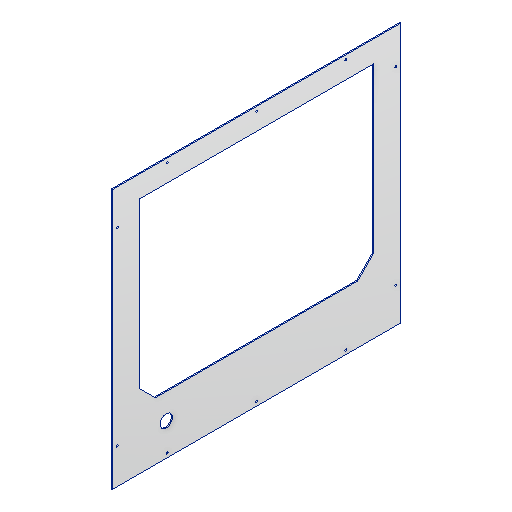
# Autodesk Inventor part: Front Panel
Saved by Autodesk Inventor 2023.2 (Build 272271000, 271)
## iProperties
Created: 2023-02-06
Part Number: Front Panel
Material: Aluminum 6061
Document SubType Name: Modeling
Designer: remop
Density: 2.7 g/cm^3
Appearance: Aluminum - Flat
Author: remop
Autodesk Inventor part; units mm, degrees
ref_plane "YZ Plane" through (0, 0, 0) normal (1, 0, 0) x (0, 1, 0)
ref_plane "XZ Plane" through (0, 0, 0) normal (0, 1, 0) x (-1, 0, 0)
ref_plane "XY Plane" through (0, 0, 0) normal (0, 0, 1) x (1, 0, 0)
sketch "Sketch1" plane through (0, 0, 0) normal (1, 0, 0) x (0, 1, 0)
  line L0 (465, 411) -> (465, -123) projected
  line L1 (465, -123) -> (-15, -123) projected
  line L2 (-15, -123) -> (-15, 411) projected
  line L3 (-15, 411) -> (465, 411) projected
  circle A0 centre (400, -113.5) radius 1.75 projected
  circle A1 centre (50, 401.5) radius 1.75 projected
  circle A2 centre (400, 401.5) radius 1.75 projected
  circle A3 centre (-7.5, -21) radius 1.75 projected
  circle A4 centre (-7.5, 144) radius 1.75 projected
  circle A5 centre (-7.5, 309) radius 1.75 projected
  circle A6 centre (457.5, 144) radius 1.75 projected
  circle A7 centre (457.5, -21) radius 1.75 projected
  circle A8 centre (457.5, 309) radius 1.75 projected
  circle A9 centre (50, -113.5) radius 1.75 projected
  circle A10 centre (408.5, -78.0001) radius 1.75 projected
  circle A11 centre (415.5, -88.0001) radius 1.75 projected
  circle A12 centre (408.5, -88.0001) radius 1.75 projected
  circle A13 centre (415.5, -78.0001) radius 1.75 projected
  line L4 (32, 375.1132) -> (32, 380.8868) projected
  line L5 (32, 380.8868) -> (27, 383.7735) projected
  line L6 (27, 383.7735) -> (22, 380.8868) projected
  line L7 (22, 380.8868) -> (22, 375.1132) projected
  line L8 (22, 375.1132) -> (27, 372.2265) projected
  line L9 (27, 372.2265) -> (32, 375.1132) projected
  line L10 (44.5, 367.8964) -> (44.5, 362.1229) projected
  line L11 (44.5, 362.1229) -> (49.5, 359.2361) projected
  line L12 (49.5, 359.2361) -> (54.5, 362.1229) projected
  line L13 (54.5, 362.1229) -> (54.5, 367.8964) projected
  line L14 (54.5, 367.8964) -> (49.5, 370.7831) projected
  line L15 (49.5, 370.7831) -> (44.5, 367.8964) projected
  line L16 (39.5, 336.1229) -> (39.5, 341.8964) projected
  line L17 (39.5, 341.8964) -> (34.5, 344.7831) projected
  line L18 (34.5, 344.7831) -> (29.5, 341.8964) projected
  line L19 (29.5, 341.8964) -> (29.5, 336.1229) projected
  line L20 (29.5, 336.1229) -> (34.5, 333.2361) projected
  line L21 (34.5, 333.2361) -> (39.5, 336.1229) projected
  line L22 (12, 331.7735) -> (7, 328.8868) projected
  line L23 (7, 328.8868) -> (7, 323.1132) projected
  line L24 (7, 323.1132) -> (12, 320.2265) projected
  line L25 (12, 320.2265) -> (17, 323.1132) projected
  line L26 (17, 323.1132) -> (17, 328.8868) projected
  line L27 (17, 328.8868) -> (12, 331.7735) projected
  line L28 (54.5, 315.8964) -> (49.5, 318.7831) projected
  line L29 (49.5, 318.7831) -> (44.5, 315.8964) projected
  line L30 (44.5, 315.8964) -> (44.5, 310.1229) projected
  line L31 (44.5, 310.1229) -> (49.5, 307.2361) projected
  line L32 (49.5, 307.2361) -> (54.5, 310.1229) projected
  line L33 (54.5, 310.1229) -> (54.5, 315.8964) projected
  line L34 (14.5, 310.1229) -> (19.5, 307.2361) projected
  line L35 (19.5, 307.2361) -> (24.5, 310.1229) projected
  line L36 (24.5, 310.1229) -> (24.5, 315.8964) projected
  line L37 (24.5, 315.8964) -> (19.5, 318.7831) projected
  line L38 (19.5, 318.7831) -> (14.5, 315.8964) projected
  line L39 (14.5, 315.8964) -> (14.5, 310.1229) projected
  line L40 (14.5, 284.1229) -> (19.5, 281.2361) projected
  line L41 (19.5, 281.2361) -> (24.5, 284.1229) projected
  line L42 (24.5, 284.1229) -> (24.5, 289.8964) projected
  line L43 (24.5, 289.8964) -> (19.5, 292.7831) projected
  line L44 (19.5, 292.7831) -> (14.5, 289.8964) projected
  line L45 (14.5, 289.8964) -> (14.5, 284.1229) projected
  line L46 (32, 276.8868) -> (27, 279.7735) projected
  line L47 (27, 279.7735) -> (22, 276.8868) projected
  line L48 (22, 276.8868) -> (22, 271.1132) projected
  line L49 (22, 271.1132) -> (27, 268.2265) projected
  line L50 (27, 268.2265) -> (32, 271.1132) projected
  line L51 (32, 271.1132) -> (32, 276.8868) projected
  line L52 (54.5, 263.8964) -> (49.5, 266.7831) projected
  line L53 (49.5, 266.7831) -> (44.5, 263.8964) projected
  line L54 (44.5, 263.8964) -> (44.5, 258.1229) projected
  line L55 (44.5, 258.1229) -> (49.5, 255.2361) projected
  line L56 (49.5, 255.2361) -> (54.5, 258.1229) projected
  line L57 (54.5, 258.1229) -> (54.5, 263.8964) projected
  line L58 (12, 253.7735) -> (7, 250.8868) projected
  line L59 (7, 250.8868) -> (7, 245.1132) projected
  line L60 (7, 245.1132) -> (12, 242.2265) projected
  line L61 (12, 242.2265) -> (17, 245.1132) projected
  line L62 (17, 245.1132) -> (17, 250.8868) projected
  line L63 (17, 250.8868) -> (12, 253.7735) projected
  line L64 (32, 224.8868) -> (27, 227.7735) projected
  line L65 (27, 227.7735) -> (22, 224.8868) projected
  line L66 (22, 224.8868) -> (22, 219.1132) projected
  line L67 (22, 219.1132) -> (27, 216.2265) projected
  line L68 (27, 216.2265) -> (32, 219.1132) projected
  line L69 (32, 219.1132) -> (32, 224.8868) projected
  line L70 (57, 227.7735) -> (52, 224.8868) projected
  line L71 (52, 224.8868) -> (52, 219.1132) projected
  line L72 (52, 219.1132) -> (57, 216.2265) projected
  line L73 (57, 216.2265) -> (62, 219.1132) projected
  line L74 (62, 219.1132) -> (62, 224.8868) projected
  line L75 (62, 224.8868) -> (57, 227.7735) projected
  line L76 (54.5, 185.8964) -> (49.5, 188.7831) projected
  line L77 (49.5, 188.7831) -> (44.5, 185.8964) projected
  line L78 (44.5, 185.8964) -> (44.5, 180.1229) projected
  line L79 (44.5, 180.1229) -> (49.5, 177.2361) projected
  line L80 (49.5, 177.2361) -> (54.5, 180.1229) projected
  line L81 (54.5, 180.1229) -> (54.5, 185.8964) projected
  line L82 (32, 198.8868) -> (27, 201.7735) projected
  line L83 (27, 201.7735) -> (22, 198.8868) projected
  line L84 (22, 198.8868) -> (22, 193.1132) projected
  line L85 (22, 193.1132) -> (27, 190.2265) projected
  line L86 (27, 190.2265) -> (32, 193.1132) projected
  line L87 (32, 193.1132) -> (32, 198.8868) projected
  line L88 (32, 172.8868) -> (27, 175.7735) projected
  line L89 (27, 175.7735) -> (22, 172.8868) projected
  line L90 (22, 172.8868) -> (22, 167.1132) projected
  line L91 (22, 167.1132) -> (27, 164.2265) projected
  line L92 (27, 164.2265) -> (32, 167.1132) projected
  line L93 (32, 167.1132) -> (32, 172.8868) projected
  line L94 (54.5, 159.8964) -> (49.5, 162.7831) projected
  line L95 (49.5, 162.7831) -> (44.5, 159.8964) projected
  line L96 (44.5, 159.8964) -> (44.5, 154.1229) projected
  line L97 (44.5, 154.1229) -> (49.5, 151.2361) projected
  line L98 (49.5, 151.2361) -> (54.5, 154.1229) projected
  line L99 (54.5, 154.1229) -> (54.5, 159.8964) projected
  line L100 (39.5, 128.1229) -> (39.5, 133.8964) projected
  line L101 (39.5, 133.8964) -> (34.5, 136.7831) projected
  line L102 (34.5, 136.7831) -> (29.5, 133.8964) projected
  line L103 (29.5, 133.8964) -> (29.5, 128.1229) projected
  line L104 (29.5, 128.1229) -> (34.5, 125.2361) projected
  line L105 (34.5, 125.2361) -> (39.5, 128.1229) projected
  line L106 (12, 123.7735) -> (7, 120.8868) projected
  line L107 (7, 120.8868) -> (7, 115.1132) projected
  line L108 (7, 115.1132) -> (12, 112.2265) projected
  line L109 (12, 112.2265) -> (17, 115.1132) projected
  line L110 (17, 115.1132) -> (17, 120.8868) projected
  line L111 (17, 120.8868) -> (12, 123.7735) projected
  line L112 (54.5, 107.8964) -> (49.5, 110.7831) projected
  line L113 (49.5, 110.7831) -> (44.5, 107.8964) projected
  line L114 (44.5, 107.8964) -> (44.5, 102.1229) projected
  line L115 (44.5, 102.1229) -> (49.5, 99.2361) projected
  line L116 (49.5, 99.2361) -> (54.5, 102.1229) projected
  line L117 (54.5, 102.1229) -> (54.5, 107.8964) projected
  line L118 (14.5, 102.1229) -> (19.5, 99.2361) projected
  line L119 (19.5, 99.2361) -> (24.5, 102.1229) projected
  line L120 (24.5, 102.1229) -> (24.5, 107.8964) projected
  line L121 (24.5, 107.8964) -> (19.5, 110.7831) projected
  line L122 (19.5, 110.7831) -> (14.5, 107.8964) projected
  line L123 (14.5, 107.8964) -> (14.5, 102.1229) projected
  line L124 (39.5, 76.1229) -> (39.5, 81.8964) projected
  line L125 (39.5, 81.8964) -> (34.5, 84.7831) projected
  line L126 (34.5, 84.7831) -> (29.5, 81.8964) projected
  line L127 (29.5, 81.8964) -> (29.5, 76.1229) projected
  line L128 (29.5, 76.1229) -> (34.5, 73.2361) projected
  line L129 (34.5, 73.2361) -> (39.5, 76.1229) projected
  line L130 (42, 71.7735) -> (37, 68.8868) projected
  line L131 (37, 68.8868) -> (37, 63.1132) projected
  line L132 (37, 63.1132) -> (42, 60.2265) projected
  line L133 (42, 60.2265) -> (47, 63.1132) projected
  line L134 (47, 63.1132) -> (47, 68.8868) projected
  line L135 (47, 68.8868) -> (42, 71.7735) projected
  line L136 (14.5, 50.1229) -> (19.5, 47.2361) projected
  line L137 (19.5, 47.2361) -> (24.5, 50.1229) projected
  line L138 (24.5, 50.1229) -> (24.5, 55.8964) projected
  line L139 (24.5, 55.8964) -> (19.5, 58.7831) projected
  line L140 (19.5, 58.7831) -> (14.5, 55.8964) projected
  line L141 (14.5, 55.8964) -> (14.5, 50.1229) projected
  line L142 (12, 45.7735) -> (7, 42.8868) projected
  line L143 (7, 42.8868) -> (7, 37.1132) projected
  line L144 (7, 37.1132) -> (12, 34.2265) projected
  line L145 (12, 34.2265) -> (17, 37.1132) projected
  line L146 (17, 37.1132) -> (17, 42.8868) projected
  line L147 (17, 42.8868) -> (12, 45.7735) projected
  line L148 (57, 19.7735) -> (52, 16.8868) projected
  line L149 (52, 16.8868) -> (52, 11.1132) projected
  line L150 (52, 11.1132) -> (57, 8.2265) projected
  line L151 (57, 8.2265) -> (62, 11.1132) projected
  line L152 (62, 11.1132) -> (62, 16.8868) projected
  line L153 (62, 16.8868) -> (57, 19.7735) projected
  line L154 (39.5, -1.8771) -> (39.5, 3.8964) projected
  line L155 (39.5, 3.8964) -> (34.5, 6.7831) projected
  line L156 (34.5, 6.7831) -> (29.5, 3.8964) projected
  line L157 (29.5, 3.8964) -> (29.5, -1.8771) projected
  line L158 (29.5, -1.8771) -> (34.5, -4.7639) projected
  line L159 (34.5, -4.7639) -> (39.5, -1.8771) projected
  line L160 (14.5, -1.8771) -> (19.5, -4.7639) projected
  line L161 (19.5, -4.7639) -> (24.5, -1.8771) projected
  line L162 (24.5, -1.8771) -> (24.5, 3.8964) projected
  line L163 (24.5, 3.8964) -> (19.5, 6.7831) projected
  line L164 (19.5, 6.7831) -> (14.5, 3.8964) projected
  line L165 (14.5, 3.8964) -> (14.5, -1.8771) projected
  line L166 (39.5, -27.8771) -> (39.5, -22.1036) projected
  line L167 (39.5, -22.1036) -> (34.5, -19.2169) projected
  line L168 (34.5, -19.2169) -> (29.5, -22.1036) projected
  line L169 (29.5, -22.1036) -> (29.5, -27.8771) projected
  line L170 (29.5, -27.8771) -> (34.5, -30.7639) projected
  line L171 (34.5, -30.7639) -> (39.5, -27.8771) projected
  line L172 (32, -35.1132) -> (27, -32.2265) projected
  line L173 (27, -32.2265) -> (22, -35.1132) projected
  line L174 (22, -35.1132) -> (22, -40.8868) projected
  line L175 (22, -40.8868) -> (27, -43.7735) projected
  line L176 (27, -43.7735) -> (32, -40.8868) projected
  line L177 (32, -40.8868) -> (32, -35.1132) projected
  line L178 (54.5, -48.1036) -> (49.5, -45.2169) projected
  line L179 (49.5, -45.2169) -> (44.5, -48.1036) projected
  line L180 (44.5, -48.1036) -> (44.5, -53.8771) projected
  line L181 (44.5, -53.8771) -> (49.5, -56.7639) projected
  line L182 (49.5, -56.7639) -> (54.5, -53.8771) projected
  line L183 (54.5, -53.8771) -> (54.5, -48.1036) projected
  line L184 (12, -58.2265) -> (7, -61.1132) projected
  line L185 (7, -61.1132) -> (7, -66.8868) projected
  line L186 (7, -66.8868) -> (12, -69.7735) projected
  line L187 (12, -69.7735) -> (17, -66.8868) projected
  line L188 (17, -66.8868) -> (17, -61.1132) projected
  line L189 (17, -61.1132) -> (12, -58.2265) projected
  line L190 (57, -84.2265) -> (52, -87.1132) projected
  line L191 (52, -87.1132) -> (52, -92.8868) projected
  line L192 (52, -92.8868) -> (57, -95.7735) projected
  line L193 (57, -95.7735) -> (62, -92.8868) projected
  line L194 (62, -92.8868) -> (62, -87.1132) projected
  line L195 (62, -87.1132) -> (57, -84.2265) projected
  line L196 (12, -84.2265) -> (7, -87.1132) projected
  line L197 (7, -87.1132) -> (7, -92.8868) projected
  line L198 (7, -92.8868) -> (12, -95.7735) projected
  line L199 (12, -95.7735) -> (17, -92.8868) projected
  line L200 (17, -92.8868) -> (17, -87.1132) projected
  line L201 (17, -87.1132) -> (12, -84.2265) projected
  line L202 (54.5, -74.1036) -> (49.5, -71.2169) projected
  line L203 (49.5, -71.2169) -> (44.5, -74.1036) projected
  line L204 (44.5, -74.1036) -> (44.5, -79.8771) projected
  line L205 (44.5, -79.8771) -> (49.5, -82.7639) projected
  line L206 (49.5, -82.7639) -> (54.5, -79.8771) projected
  line L207 (54.5, -79.8771) -> (54.5, -74.1036) projected
  line L208 (32, -61.1132) -> (27, -58.2265) projected
  line L209 (27, -58.2265) -> (22, -61.1132) projected
  line L210 (22, -61.1132) -> (22, -66.8868) projected
  line L211 (22, -66.8868) -> (27, -69.7735) projected
  line L212 (27, -69.7735) -> (32, -66.8868) projected
  line L213 (32, -66.8868) -> (32, -61.1132) projected
  line L214 (39.5, -53.8771) -> (39.5, -48.1036) projected
  line L215 (39.5, -48.1036) -> (34.5, -45.2169) projected
  line L216 (34.5, -45.2169) -> (29.5, -48.1036) projected
  line L217 (29.5, -48.1036) -> (29.5, -53.8771) projected
  line L218 (29.5, -53.8771) -> (34.5, -56.7639) projected
  line L219 (34.5, -56.7639) -> (39.5, -53.8771) projected
  line L220 (42, -32.2265) -> (37, -35.1132) projected
  line L221 (37, -35.1132) -> (37, -40.8868) projected
  line L222 (37, -40.8868) -> (42, -43.7735) projected
  line L223 (42, -43.7735) -> (47, -40.8868) projected
  line L224 (47, -40.8868) -> (47, -35.1132) projected
  line L225 (47, -35.1132) -> (42, -32.2265) projected
  line L226 (14.5, -27.8771) -> (19.5, -30.7639) projected
  line L227 (19.5, -30.7639) -> (24.5, -27.8771) projected
  line L228 (24.5, -27.8771) -> (24.5, -22.1036) projected
  line L229 (24.5, -22.1036) -> (19.5, -19.2169) projected
  line L230 (19.5, -19.2169) -> (14.5, -22.1036) projected
  line L231 (14.5, -22.1036) -> (14.5, -27.8771) projected
  line L232 (12, 19.7735) -> (7, 16.8868) projected
  line L233 (7, 16.8868) -> (7, 11.1132) projected
  line L234 (7, 11.1132) -> (12, 8.2265) projected
  line L235 (12, 8.2265) -> (17, 11.1132) projected
  line L236 (17, 11.1132) -> (17, 16.8868) projected
  line L237 (17, 16.8868) -> (12, 19.7735) projected
  line L238 (42, -6.2265) -> (37, -9.1132) projected
  line L239 (37, -9.1132) -> (37, -14.8868) projected
  line L240 (37, -14.8868) -> (42, -17.7735) projected
  line L241 (42, -17.7735) -> (47, -14.8868) projected
  line L242 (47, -14.8868) -> (47, -9.1132) projected
  line L243 (47, -9.1132) -> (42, -6.2265) projected
  line L244 (54.5, 29.8964) -> (49.5, 32.7831) projected
  line L245 (49.5, 32.7831) -> (44.5, 29.8964) projected
  line L246 (44.5, 29.8964) -> (44.5, 24.1229) projected
  line L247 (44.5, 24.1229) -> (49.5, 21.2361) projected
  line L248 (49.5, 21.2361) -> (54.5, 24.1229) projected
  line L249 (54.5, 24.1229) -> (54.5, 29.8964) projected
  line L250 (32, 42.8868) -> (27, 45.7735) projected
  line L251 (27, 45.7735) -> (22, 42.8868) projected
  line L252 (22, 42.8868) -> (22, 37.1132) projected
  line L253 (22, 37.1132) -> (27, 34.2265) projected
  line L254 (27, 34.2265) -> (32, 37.1132) projected
  line L255 (32, 37.1132) -> (32, 42.8868) projected
  line L256 (12, 71.7735) -> (7, 68.8868) projected
  line L257 (7, 68.8868) -> (7, 63.1132) projected
  line L258 (7, 63.1132) -> (12, 60.2265) projected
  line L259 (12, 60.2265) -> (17, 63.1132) projected
  line L260 (17, 63.1132) -> (17, 68.8868) projected
  line L261 (17, 68.8868) -> (12, 71.7735) projected
  line L262 (54.5, 55.8964) -> (49.5, 58.7831) projected
  line L263 (49.5, 58.7831) -> (44.5, 55.8964) projected
  line L264 (44.5, 55.8964) -> (44.5, 50.1229) projected
  line L265 (44.5, 50.1229) -> (49.5, 47.2361) projected
  line L266 (49.5, 47.2361) -> (54.5, 50.1229) projected
  line L267 (54.5, 50.1229) -> (54.5, 55.8964) projected
  line L268 (14.5, 76.1229) -> (19.5, 73.2361) projected
  line L269 (19.5, 73.2361) -> (24.5, 76.1229) projected
  line L270 (24.5, 76.1229) -> (24.5, 81.8964) projected
  line L271 (24.5, 81.8964) -> (19.5, 84.7831) projected
  line L272 (19.5, 84.7831) -> (14.5, 81.8964) projected
  line L273 (14.5, 81.8964) -> (14.5, 76.1229) projected
  line L274 (39.5, 102.1229) -> (39.5, 107.8964) projected
  line L275 (39.5, 107.8964) -> (34.5, 110.7831) projected
  line L276 (34.5, 110.7831) -> (29.5, 107.8964) projected
  line L277 (29.5, 107.8964) -> (29.5, 102.1229) projected
  line L278 (29.5, 102.1229) -> (34.5, 99.2361) projected
  line L279 (34.5, 99.2361) -> (39.5, 102.1229) projected
  line L280 (57, 123.7735) -> (52, 120.8868) projected
  line L281 (52, 120.8868) -> (52, 115.1132) projected
  line L282 (52, 115.1132) -> (57, 112.2265) projected
  line L283 (57, 112.2265) -> (62, 115.1132) projected
  line L284 (62, 115.1132) -> (62, 120.8868) projected
  line L285 (62, 120.8868) -> (57, 123.7735) projected
  line L286 (14.5, 128.1229) -> (19.5, 125.2361) projected
  line L287 (19.5, 125.2361) -> (24.5, 128.1229) projected
  line L288 (24.5, 128.1229) -> (24.5, 133.8964) projected
  line L289 (24.5, 133.8964) -> (19.5, 136.7831) projected
  line L290 (19.5, 136.7831) -> (14.5, 133.8964) projected
  line L291 (14.5, 133.8964) -> (14.5, 128.1229) projected
  line L292 (42, 149.7735) -> (37, 146.8868) projected
  line L293 (37, 146.8868) -> (37, 141.1132) projected
  line L294 (37, 141.1132) -> (42, 138.2265) projected
  line L295 (42, 138.2265) -> (47, 141.1132) projected
  line L296 (47, 141.1132) -> (47, 146.8868) projected
  line L297 (47, 146.8868) -> (42, 149.7735) projected
  line L298 (39.5, 154.1229) -> (39.5, 159.8964) projected
  line L299 (39.5, 159.8964) -> (34.5, 162.7831) projected
  line L300 (34.5, 162.7831) -> (29.5, 159.8964) projected
  line L301 (29.5, 159.8964) -> (29.5, 154.1229) projected
  line L302 (29.5, 154.1229) -> (34.5, 151.2361) projected
  line L303 (34.5, 151.2361) -> (39.5, 154.1229) projected
  line L304 (12, 201.7735) -> (7, 198.8868) projected
  line L305 (7, 198.8868) -> (7, 193.1132) projected
  line L306 (7, 193.1132) -> (12, 190.2265) projected
  line L307 (12, 190.2265) -> (17, 193.1132) projected
  line L308 (17, 193.1132) -> (17, 198.8868) projected
  line L309 (17, 198.8868) -> (12, 201.7735) projected
  line L310 (39.5, 180.1229) -> (39.5, 185.8964) projected
  line L311 (39.5, 185.8964) -> (34.5, 188.7831) projected
  line L312 (34.5, 188.7831) -> (29.5, 185.8964) projected
  line L313 (29.5, 185.8964) -> (29.5, 180.1229) projected
  line L314 (29.5, 180.1229) -> (34.5, 177.2361) projected
  line L315 (34.5, 177.2361) -> (39.5, 180.1229) projected
  line L316 (57, 201.7735) -> (52, 198.8868) projected
  line L317 (52, 198.8868) -> (52, 193.1132) projected
  line L318 (52, 193.1132) -> (57, 190.2265) projected
  line L319 (57, 190.2265) -> (62, 193.1132) projected
  line L320 (62, 193.1132) -> (62, 198.8868) projected
  line L321 (62, 198.8868) -> (57, 201.7735) projected
  line L322 (42, 227.7735) -> (37, 224.8868) projected
  line L323 (37, 224.8868) -> (37, 219.1132) projected
  line L324 (37, 219.1132) -> (42, 216.2265) projected
  line L325 (42, 216.2265) -> (47, 219.1132) projected
  line L326 (47, 219.1132) -> (47, 224.8868) projected
  line L327 (47, 224.8868) -> (42, 227.7735) projected
  line L328 (14.5, 232.1229) -> (19.5, 229.2361) projected
  line L329 (19.5, 229.2361) -> (24.5, 232.1229) projected
  line L330 (24.5, 232.1229) -> (24.5, 237.8964) projected
  line L331 (24.5, 237.8964) -> (19.5, 240.7831) projected
  line L332 (19.5, 240.7831) -> (14.5, 237.8964) projected
  line L333 (14.5, 237.8964) -> (14.5, 232.1229) projected
  line L334 (32, 250.8868) -> (27, 253.7735) projected
  line L335 (27, 253.7735) -> (22, 250.8868) projected
  line L336 (22, 250.8868) -> (22, 245.1132) projected
  line L337 (22, 245.1132) -> (27, 242.2265) projected
  line L338 (27, 242.2265) -> (32, 245.1132) projected
  line L339 (32, 245.1132) -> (32, 250.8868) projected
  line L340 (39.5, 258.1229) -> (39.5, 263.8964) projected
  line L341 (39.5, 263.8964) -> (34.5, 266.7831) projected
  line L342 (34.5, 266.7831) -> (29.5, 263.8964) projected
  line L343 (29.5, 263.8964) -> (29.5, 258.1229) projected
  line L344 (29.5, 258.1229) -> (34.5, 255.2361) projected
  line L345 (34.5, 255.2361) -> (39.5, 258.1229) projected
  line L346 (42, 279.7735) -> (37, 276.8868) projected
  line L347 (37, 276.8868) -> (37, 271.1132) projected
  line L348 (37, 271.1132) -> (42, 268.2265) projected
  line L349 (42, 268.2265) -> (47, 271.1132) projected
  line L350 (47, 271.1132) -> (47, 276.8868) projected
  line L351 (47, 276.8868) -> (42, 279.7735) projected
  line L352 (39.5, 284.1229) -> (39.5, 289.8964) projected
  line L353 (39.5, 289.8964) -> (34.5, 292.7831) projected
  line L354 (34.5, 292.7831) -> (29.5, 289.8964) projected
  line L355 (29.5, 289.8964) -> (29.5, 284.1229) projected
  line L356 (29.5, 284.1229) -> (34.5, 281.2361) projected
  line L357 (34.5, 281.2361) -> (39.5, 284.1229) projected
  line L358 (39.5, 310.1229) -> (39.5, 315.8964) projected
  line L359 (39.5, 315.8964) -> (34.5, 318.7831) projected
  line L360 (34.5, 318.7831) -> (29.5, 315.8964) projected
  line L361 (29.5, 315.8964) -> (29.5, 310.1229) projected
  line L362 (29.5, 310.1229) -> (34.5, 307.2361) projected
  line L363 (34.5, 307.2361) -> (39.5, 310.1229) projected
  line L364 (57, 331.7735) -> (52, 328.8868) projected
  line L365 (52, 328.8868) -> (52, 323.1132) projected
  line L366 (52, 323.1132) -> (57, 320.2265) projected
  line L367 (57, 320.2265) -> (62, 323.1132) projected
  line L368 (62, 323.1132) -> (62, 328.8868) projected
  line L369 (62, 328.8868) -> (57, 331.7735) projected
  line L370 (14.5, 336.1229) -> (19.5, 333.2361) projected
  line L371 (19.5, 333.2361) -> (24.5, 336.1229) projected
  line L372 (24.5, 336.1229) -> (24.5, 341.8964) projected
  line L373 (24.5, 341.8964) -> (19.5, 344.7831) projected
  line L374 (19.5, 344.7831) -> (14.5, 341.8964) projected
  line L375 (14.5, 341.8964) -> (14.5, 336.1229) projected
  line L376 (42, 357.7735) -> (37, 354.8868) projected
  line L377 (37, 354.8868) -> (37, 349.1132) projected
  line L378 (37, 349.1132) -> (42, 346.2265) projected
  line L379 (42, 346.2265) -> (47, 349.1132) projected
  line L380 (47, 349.1132) -> (47, 354.8868) projected
  line L381 (47, 354.8868) -> (42, 357.7735) projected
  line L382 (29.5, 367.8964) -> (29.5, 362.1229) projected
  line L383 (29.5, 362.1229) -> (34.5, 359.2361) projected
  line L384 (34.5, 359.2361) -> (39.5, 362.1229) projected
  line L385 (39.5, 362.1229) -> (39.5, 367.8964) projected
  line L386 (39.5, 367.8964) -> (34.5, 370.7831) projected
  line L387 (34.5, 370.7831) -> (29.5, 367.8964) projected
  line L388 (47, 380.8868) -> (42, 383.7735) projected
  line L389 (42, 383.7735) -> (37, 380.8868) projected
  line L390 (37, 380.8868) -> (37, 375.1132) projected
  line L391 (37, 375.1132) -> (42, 372.2265) projected
  line L392 (42, 372.2265) -> (47, 375.1132) projected
  line L393 (47, 375.1132) -> (47, 380.8868) projected
  line L394 (17, 380.8868) -> (12, 383.7735) projected
  line L395 (12, 383.7735) -> (7, 380.8868) projected
  line L396 (7, 380.8868) -> (7, 375.1132) projected
  line L397 (7, 375.1132) -> (12, 372.2265) projected
  line L398 (12, 372.2265) -> (17, 375.1132) projected
  line L399 (17, 375.1132) -> (17, 380.8868) projected
  line L400 (57, 357.7735) -> (52, 354.8868) projected
  line L401 (52, 354.8868) -> (52, 349.1132) projected
  line L402 (52, 349.1132) -> (57, 346.2265) projected
  line L403 (57, 346.2265) -> (62, 349.1132) projected
  line L404 (62, 349.1132) -> (62, 354.8868) projected
  line L405 (62, 354.8868) -> (57, 357.7735) projected
  line L406 (32, 354.8868) -> (27, 357.7735) projected
  line L407 (27, 357.7735) -> (22, 354.8868) projected
  line L408 (22, 354.8868) -> (22, 349.1132) projected
  line L409 (22, 349.1132) -> (27, 346.2265) projected
  line L410 (27, 346.2265) -> (32, 349.1132) projected
  line L411 (32, 349.1132) -> (32, 354.8868) projected
  line L412 (32, 328.8868) -> (27, 331.7735) projected
  line L413 (27, 331.7735) -> (22, 328.8868) projected
  line L414 (22, 328.8868) -> (22, 323.1132) projected
  line L415 (22, 323.1132) -> (27, 320.2265) projected
  line L416 (27, 320.2265) -> (32, 323.1132) projected
  line L417 (32, 323.1132) -> (32, 328.8868) projected
  line L418 (57, 305.7735) -> (52, 302.8868) projected
  line L419 (52, 302.8868) -> (52, 297.1132) projected
  line L420 (52, 297.1132) -> (57, 294.2265) projected
  line L421 (57, 294.2265) -> (62, 297.1132) projected
  line L422 (62, 297.1132) -> (62, 302.8868) projected
  line L423 (62, 302.8868) -> (57, 305.7735) projected
  line L424 (12, 305.7735) -> (7, 302.8868) projected
  line L425 (7, 302.8868) -> (7, 297.1132) projected
  line L426 (7, 297.1132) -> (12, 294.2265) projected
  line L427 (12, 294.2265) -> (17, 297.1132) projected
  line L428 (17, 297.1132) -> (17, 302.8868) projected
  line L429 (17, 302.8868) -> (12, 305.7735) projected
  line L430 (54.5, 289.8964) -> (49.5, 292.7831) projected
  line L431 (49.5, 292.7831) -> (44.5, 289.8964) projected
  line L432 (44.5, 289.8964) -> (44.5, 284.1229) projected
  line L433 (44.5, 284.1229) -> (49.5, 281.2361) projected
  line L434 (49.5, 281.2361) -> (54.5, 284.1229) projected
  line L435 (54.5, 284.1229) -> (54.5, 289.8964) projected
  line L436 (12, 279.7735) -> (7, 276.8868) projected
  line L437 (7, 276.8868) -> (7, 271.1132) projected
  line L438 (7, 271.1132) -> (12, 268.2265) projected
  line L439 (12, 268.2265) -> (17, 271.1132) projected
  line L440 (17, 271.1132) -> (17, 276.8868) projected
  line L441 (17, 276.8868) -> (12, 279.7735) projected
  line L442 (57, 253.7735) -> (52, 250.8868) projected
  line L443 (52, 250.8868) -> (52, 245.1132) projected
  line L444 (52, 245.1132) -> (57, 242.2265) projected
  line L445 (57, 242.2265) -> (62, 245.1132) projected
  line L446 (62, 245.1132) -> (62, 250.8868) projected
  line L447 (62, 250.8868) -> (57, 253.7735) projected
  line L448 (54.5, 237.8964) -> (49.5, 240.7831) projected
  line L449 (49.5, 240.7831) -> (44.5, 237.8964) projected
  line L450 (44.5, 237.8964) -> (44.5, 232.1229) projected
  line L451 (44.5, 232.1229) -> (49.5, 229.2361) projected
  line L452 (49.5, 229.2361) -> (54.5, 232.1229) projected
  line L453 (54.5, 232.1229) -> (54.5, 237.8964) projected
  line L454 (14.5, 206.1229) -> (19.5, 203.2361) projected
  line L455 (19.5, 203.2361) -> (24.5, 206.1229) projected
  line L456 (24.5, 206.1229) -> (24.5, 211.8964) projected
  line L457 (24.5, 211.8964) -> (19.5, 214.7831) projected
  line L458 (19.5, 214.7831) -> (14.5, 211.8964) projected
  line L459 (14.5, 211.8964) -> (14.5, 206.1229) projected
  line L460 (54.5, 211.8964) -> (49.5, 214.7831) projected
  line L461 (49.5, 214.7831) -> (44.5, 211.8964) projected
  line L462 (44.5, 211.8964) -> (44.5, 206.1229) projected
  line L463 (44.5, 206.1229) -> (49.5, 203.2361) projected
  line L464 (49.5, 203.2361) -> (54.5, 206.1229) projected
  line L465 (54.5, 206.1229) -> (54.5, 211.8964) projected
  line L466 (57, 175.7735) -> (52, 172.8868) projected
  line L467 (52, 172.8868) -> (52, 167.1132) projected
  line L468 (52, 167.1132) -> (57, 164.2265) projected
  line L469 (57, 164.2265) -> (62, 167.1132) projected
  line L470 (62, 167.1132) -> (62, 172.8868) projected
  line L471 (62, 172.8868) -> (57, 175.7735) projected
  line L472 (42, 201.7735) -> (37, 198.8868) projected
  line L473 (37, 198.8868) -> (37, 193.1132) projected
  line L474 (37, 193.1132) -> (42, 190.2265) projected
  line L475 (42, 190.2265) -> (47, 193.1132) projected
  line L476 (47, 193.1132) -> (47, 198.8868) projected
  line L477 (47, 198.8868) -> (42, 201.7735) projected
  line L478 (12, 175.7735) -> (7, 172.8868) projected
  line L479 (7, 172.8868) -> (7, 167.1132) projected
  line L480 (7, 167.1132) -> (12, 164.2265) projected
  line L481 (12, 164.2265) -> (17, 167.1132) projected
  line L482 (17, 167.1132) -> (17, 172.8868) projected
  line L483 (17, 172.8868) -> (12, 175.7735) projected
  line L484 (57, 149.7735) -> (52, 146.8868) projected
  line L485 (52, 146.8868) -> (52, 141.1132) projected
  line L486 (52, 141.1132) -> (57, 138.2265) projected
  line L487 (57, 138.2265) -> (62, 141.1132) projected
  line L488 (62, 141.1132) -> (62, 146.8868) projected
  line L489 (62, 146.8868) -> (57, 149.7735) projected
  line L490 (32, 146.8868) -> (27, 149.7735) projected
  line L491 (27, 149.7735) -> (22, 146.8868) projected
  line L492 (22, 146.8868) -> (22, 141.1132) projected
  line L493 (22, 141.1132) -> (27, 138.2265) projected
  line L494 (27, 138.2265) -> (32, 141.1132) projected
  line L495 (32, 141.1132) -> (32, 146.8868) projected
  line L496 (32, 120.8868) -> (27, 123.7735) projected
  line L497 (27, 123.7735) -> (22, 120.8868) projected
  line L498 (22, 120.8868) -> (22, 115.1132) projected
  line L499 (22, 115.1132) -> (27, 112.2265) projected
  line L500 (27, 112.2265) -> (32, 115.1132) projected
  line L501 (32, 115.1132) -> (32, 120.8868) projected
  line L502 (57, 97.7735) -> (52, 94.8868) projected
  line L503 (52, 94.8868) -> (52, 89.1132) projected
  line L504 (52, 89.1132) -> (57, 86.2265) projected
  line L505 (57, 86.2265) -> (62, 89.1132) projected
  line L506 (62, 89.1132) -> (62, 94.8868) projected
  line L507 (62, 94.8868) -> (57, 97.7735) projected
  line L508 (32, 94.8868) -> (27, 97.7735) projected
  line L509 (27, 97.7735) -> (22, 94.8868) projected
  line L510 (22, 94.8868) -> (22, 89.1132) projected
  line L511 (22, 89.1132) -> (27, 86.2265) projected
  line L512 (27, 86.2265) -> (32, 89.1132) projected
  line L513 (32, 89.1132) -> (32, 94.8868) projected
  line L514 (54.5, 81.8964) -> (49.5, 84.7831) projected
  line L515 (49.5, 84.7831) -> (44.5, 81.8964) projected
  line L516 (44.5, 81.8964) -> (44.5, 76.1229) projected
  line L517 (44.5, 76.1229) -> (49.5, 73.2361) projected
  line L518 (49.5, 73.2361) -> (54.5, 76.1229) projected
  line L519 (54.5, 76.1229) -> (54.5, 81.8964) projected
  line L520 (39.5, 50.1229) -> (39.5, 55.8964) projected
  line L521 (39.5, 55.8964) -> (34.5, 58.7831) projected
  line L522 (34.5, 58.7831) -> (29.5, 55.8964) projected
  line L523 (29.5, 55.8964) -> (29.5, 50.1229) projected
  line L524 (29.5, 50.1229) -> (34.5, 47.2361) projected
  line L525 (34.5, 47.2361) -> (39.5, 50.1229) projected
  line L526 (57, 45.7735) -> (52, 42.8868) projected
  line L527 (52, 42.8868) -> (52, 37.1132) projected
  line L528 (52, 37.1132) -> (57, 34.2265) projected
  line L529 (57, 34.2265) -> (62, 37.1132) projected
  line L530 (62, 37.1132) -> (62, 42.8868) projected
  line L531 (62, 42.8868) -> (57, 45.7735) projected
  line L532 (14.5, 24.1229) -> (19.5, 21.2361) projected
  line L533 (19.5, 21.2361) -> (24.5, 24.1229) projected
  line L534 (24.5, 24.1229) -> (24.5, 29.8964) projected
  line L535 (24.5, 29.8964) -> (19.5, 32.7831) projected
  line L536 (19.5, 32.7831) -> (14.5, 29.8964) projected
  line L537 (14.5, 29.8964) -> (14.5, 24.1229) projected
  line L538 (54.5, 3.8964) -> (49.5, 6.7831) projected
  line L539 (49.5, 6.7831) -> (44.5, 3.8964) projected
  line L540 (44.5, 3.8964) -> (44.5, -1.8771) projected
  line L541 (44.5, -1.8771) -> (49.5, -4.7639) projected
  line L542 (49.5, -4.7639) -> (54.5, -1.8771) projected
  line L543 (54.5, -1.8771) -> (54.5, 3.8964) projected
  line L544 (32, 16.8868) -> (27, 19.7735) projected
  line L545 (27, 19.7735) -> (22, 16.8868) projected
  line L546 (22, 16.8868) -> (22, 11.1132) projected
  line L547 (22, 11.1132) -> (27, 8.2265) projected
  line L548 (27, 8.2265) -> (32, 11.1132) projected
  line L549 (32, 11.1132) -> (32, 16.8868) projected
  line L550 (32, -9.1132) -> (27, -6.2265) projected
  line L551 (27, -6.2265) -> (22, -9.1132) projected
  line L552 (22, -9.1132) -> (22, -14.8868) projected
  line L553 (22, -14.8868) -> (27, -17.7735) projected
  line L554 (27, -17.7735) -> (32, -14.8868) projected
  line L555 (32, -14.8868) -> (32, -9.1132) projected
  line L556 (54.5, -22.1036) -> (49.5, -19.2169) projected
  line L557 (49.5, -19.2169) -> (44.5, -22.1036) projected
  line L558 (44.5, -22.1036) -> (44.5, -27.8771) projected
  line L559 (44.5, -27.8771) -> (49.5, -30.7639) projected
  line L560 (49.5, -30.7639) -> (54.5, -27.8771) projected
  line L561 (54.5, -27.8771) -> (54.5, -22.1036) projected
  line L562 (12, -32.2265) -> (7, -35.1132) projected
  line L563 (7, -35.1132) -> (7, -40.8868) projected
  line L564 (7, -40.8868) -> (12, -43.7735) projected
  line L565 (12, -43.7735) -> (17, -40.8868) projected
  line L566 (17, -40.8868) -> (17, -35.1132) projected
  line L567 (17, -35.1132) -> (12, -32.2265) projected
  line L568 (57, -58.2265) -> (52, -61.1132) projected
  line L569 (52, -61.1132) -> (52, -66.8868) projected
  line L570 (52, -66.8868) -> (57, -69.7735) projected
  line L571 (57, -69.7735) -> (62, -66.8868) projected
  line L572 (62, -66.8868) -> (62, -61.1132) projected
  line L573 (62, -61.1132) -> (57, -58.2265) projected
  line L574 (14.5, -79.8771) -> (19.5, -82.7639) projected
  line L575 (19.5, -82.7639) -> (24.5, -79.8771) projected
  line L576 (24.5, -79.8771) -> (24.5, -74.1036) projected
  line L577 (24.5, -74.1036) -> (19.5, -71.2169) projected
  line L578 (19.5, -71.2169) -> (14.5, -74.1036) projected
  line L579 (14.5, -74.1036) -> (14.5, -79.8771) projected
  line L580 (42, -84.2265) -> (37, -87.1132) projected
  line L581 (37, -87.1132) -> (37, -92.8868) projected
  line L582 (37, -92.8868) -> (42, -95.7735) projected
  line L583 (42, -95.7735) -> (47, -92.8868) projected
  line L584 (47, -92.8868) -> (47, -87.1132) projected
  line L585 (47, -87.1132) -> (42, -84.2265) projected
  line L586 (32, -87.1132) -> (27, -84.2265) projected
  line L587 (27, -84.2265) -> (22, -87.1132) projected
  line L588 (22, -87.1132) -> (22, -92.8868) projected
  line L589 (22, -92.8868) -> (27, -95.7735) projected
  line L590 (27, -95.7735) -> (32, -92.8868) projected
  line L591 (32, -92.8868) -> (32, -87.1132) projected
  line L592 (39.5, -79.8771) -> (39.5, -74.1036) projected
  line L593 (39.5, -74.1036) -> (34.5, -71.2169) projected
  line L594 (34.5, -71.2169) -> (29.5, -74.1036) projected
  line L595 (29.5, -74.1036) -> (29.5, -79.8771) projected
  line L596 (29.5, -79.8771) -> (34.5, -82.7639) projected
  line L597 (34.5, -82.7639) -> (39.5, -79.8771) projected
  line L598 (42, -58.2265) -> (37, -61.1132) projected
  line L599 (37, -61.1132) -> (37, -66.8868) projected
  line L600 (37, -66.8868) -> (42, -69.7735) projected
  line L601 (42, -69.7735) -> (47, -66.8868) projected
  line L602 (47, -66.8868) -> (47, -61.1132) projected
  line L603 (47, -61.1132) -> (42, -58.2265) projected
  line L604 (14.5, -53.8771) -> (19.5, -56.7639) projected
  line L605 (19.5, -56.7639) -> (24.5, -53.8771) projected
  line L606 (24.5, -53.8771) -> (24.5, -48.1036) projected
  line L607 (24.5, -48.1036) -> (19.5, -45.2169) projected
  line L608 (19.5, -45.2169) -> (14.5, -48.1036) projected
  line L609 (14.5, -48.1036) -> (14.5, -53.8771) projected
  line L610 (57, -32.2265) -> (52, -35.1132) projected
  line L611 (52, -35.1132) -> (52, -40.8868) projected
  line L612 (52, -40.8868) -> (57, -43.7735) projected
  line L613 (57, -43.7735) -> (62, -40.8868) projected
  line L614 (62, -40.8868) -> (62, -35.1132) projected
  line L615 (62, -35.1132) -> (57, -32.2265) projected
  line L616 (12, -6.2265) -> (7, -9.1132) projected
  line L617 (7, -9.1132) -> (7, -14.8868) projected
  line L618 (7, -14.8868) -> (12, -17.7735) projected
  line L619 (12, -17.7735) -> (17, -14.8868) projected
  line L620 (17, -14.8868) -> (17, -9.1132) projected
  line L621 (17, -9.1132) -> (12, -6.2265) projected
  line L622 (42, 19.7735) -> (37, 16.8868) projected
  line L623 (37, 16.8868) -> (37, 11.1132) projected
  line L624 (37, 11.1132) -> (42, 8.2265) projected
  line L625 (42, 8.2265) -> (47, 11.1132) projected
  line L626 (47, 11.1132) -> (47, 16.8868) projected
  line L627 (47, 16.8868) -> (42, 19.7735) projected
  line L628 (57, -6.2265) -> (52, -9.1132) projected
  line L629 (52, -9.1132) -> (52, -14.8868) projected
  line L630 (52, -14.8868) -> (57, -17.7735) projected
  line L631 (57, -17.7735) -> (62, -14.8868) projected
  line L632 (62, -14.8868) -> (62, -9.1132) projected
  line L633 (62, -9.1132) -> (57, -6.2265) projected
  line L634 (39.5, 24.1229) -> (39.5, 29.8964) projected
  line L635 (39.5, 29.8964) -> (34.5, 32.7831) projected
  line L636 (34.5, 32.7831) -> (29.5, 29.8964) projected
  line L637 (29.5, 29.8964) -> (29.5, 24.1229) projected
  line L638 (29.5, 24.1229) -> (34.5, 21.2361) projected
  line L639 (34.5, 21.2361) -> (39.5, 24.1229) projected
  line L640 (42, 45.7735) -> (37, 42.8868) projected
  line L641 (37, 42.8868) -> (37, 37.1132) projected
  line L642 (37, 37.1132) -> (42, 34.2265) projected
  line L643 (42, 34.2265) -> (47, 37.1132) projected
  line L644 (47, 37.1132) -> (47, 42.8868) projected
  line L645 (47, 42.8868) -> (42, 45.7735) projected
  line L646 (32, 68.8868) -> (27, 71.7735) projected
  line L647 (27, 71.7735) -> (22, 68.8868) projected
  line L648 (22, 68.8868) -> (22, 63.1132) projected
  line L649 (22, 63.1132) -> (27, 60.2265) projected
  line L650 (27, 60.2265) -> (32, 63.1132) projected
  line L651 (32, 63.1132) -> (32, 68.8868) projected
  line L652 (57, 71.7735) -> (52, 68.8868) projected
  line L653 (52, 68.8868) -> (52, 63.1132) projected
  line L654 (52, 63.1132) -> (57, 60.2265) projected
  line L655 (57, 60.2265) -> (62, 63.1132) projected
  line L656 (62, 63.1132) -> (62, 68.8868) projected
  line L657 (62, 68.8868) -> (57, 71.7735) projected
  line L658 (12, 97.7735) -> (7, 94.8868) projected
  line L659 (7, 94.8868) -> (7, 89.1132) projected
  line L660 (7, 89.1132) -> (12, 86.2265) projected
  line L661 (12, 86.2265) -> (17, 89.1132) projected
  line L662 (17, 89.1132) -> (17, 94.8868) projected
  line L663 (17, 94.8868) -> (12, 97.7735) projected
  line L664 (42, 97.7735) -> (37, 94.8868) projected
  line L665 (37, 94.8868) -> (37, 89.1132) projected
  line L666 (37, 89.1132) -> (42, 86.2265) projected
  line L667 (42, 86.2265) -> (47, 89.1132) projected
  line L668 (47, 89.1132) -> (47, 94.8868) projected
  line L669 (47, 94.8868) -> (42, 97.7735) projected
  line L670 (42, 123.7735) -> (37, 120.8868) projected
  line L671 (37, 120.8868) -> (37, 115.1132) projected
  line L672 (37, 115.1132) -> (42, 112.2265) projected
  line L673 (42, 112.2265) -> (47, 115.1132) projected
  line L674 (47, 115.1132) -> (47, 120.8868) projected
  line L675 (47, 120.8868) -> (42, 123.7735) projected
  line L676 (12, 149.7735) -> (7, 146.8868) projected
  line L677 (7, 146.8868) -> (7, 141.1132) projected
  line L678 (7, 141.1132) -> (12, 138.2265) projected
  line L679 (12, 138.2265) -> (17, 141.1132) projected
  line L680 (17, 141.1132) -> (17, 146.8868) projected
  line L681 (17, 146.8868) -> (12, 149.7735) projected
  line L682 (54.5, 133.8964) -> (49.5, 136.7831) projected
  line L683 (49.5, 136.7831) -> (44.5, 133.8964) projected
  line L684 (44.5, 133.8964) -> (44.5, 128.1229) projected
  line L685 (44.5, 128.1229) -> (49.5, 125.2361) projected
  line L686 (49.5, 125.2361) -> (54.5, 128.1229) projected
  line L687 (54.5, 128.1229) -> (54.5, 133.8964) projected
  line L688 (14.5, 154.1229) -> (19.5, 151.2361) projected
  line L689 (19.5, 151.2361) -> (24.5, 154.1229) projected
  line L690 (24.5, 154.1229) -> (24.5, 159.8964) projected
  line L691 (24.5, 159.8964) -> (19.5, 162.7831) projected
  line L692 (19.5, 162.7831) -> (14.5, 159.8964) projected
  line L693 (14.5, 159.8964) -> (14.5, 154.1229) projected
  line L694 (14.5, 180.1229) -> (19.5, 177.2361) projected
  line L695 (19.5, 177.2361) -> (24.5, 180.1229) projected
  line L696 (24.5, 180.1229) -> (24.5, 185.8964) projected
  line L697 (24.5, 185.8964) -> (19.5, 188.7831) projected
  line L698 (19.5, 188.7831) -> (14.5, 185.8964) projected
  line L699 (14.5, 185.8964) -> (14.5, 180.1229) projected
  line L700 (42, 175.7735) -> (37, 172.8868) projected
  line L701 (37, 172.8868) -> (37, 167.1132) projected
  line L702 (37, 167.1132) -> (42, 164.2265) projected
  line L703 (42, 164.2265) -> (47, 167.1132) projected
  line L704 (47, 167.1132) -> (47, 172.8868) projected
  line L705 (47, 172.8868) -> (42, 175.7735) projected
  line L706 (39.5, 206.1229) -> (39.5, 211.8964) projected
  line L707 (39.5, 211.8964) -> (34.5, 214.7831) projected
  line L708 (34.5, 214.7831) -> (29.5, 211.8964) projected
  line L709 (29.5, 211.8964) -> (29.5, 206.1229) projected
  line L710 (29.5, 206.1229) -> (34.5, 203.2361) projected
  line L711 (34.5, 203.2361) -> (39.5, 206.1229) projected
  line L712 (12, 227.7735) -> (7, 224.8868) projected
  line L713 (7, 224.8868) -> (7, 219.1132) projected
  line L714 (7, 219.1132) -> (12, 216.2265) projected
  line L715 (12, 216.2265) -> (17, 219.1132) projected
  line L716 (17, 219.1132) -> (17, 224.8868) projected
  line L717 (17, 224.8868) -> (12, 227.7735) projected
  line L718 (39.5, 232.1229) -> (39.5, 237.8964) projected
  line L719 (39.5, 237.8964) -> (34.5, 240.7831) projected
  line L720 (34.5, 240.7831) -> (29.5, 237.8964) projected
  line L721 (29.5, 237.8964) -> (29.5, 232.1229) projected
  line L722 (29.5, 232.1229) -> (34.5, 229.2361) projected
  line L723 (34.5, 229.2361) -> (39.5, 232.1229) projected
  line L724 (42, 253.7735) -> (37, 250.8868) projected
  line L725 (37, 250.8868) -> (37, 245.1132) projected
  line L726 (37, 245.1132) -> (42, 242.2265) projected
  line L727 (42, 242.2265) -> (47, 245.1132) projected
  line L728 (47, 245.1132) -> (47, 250.8868) projected
  line L729 (47, 250.8868) -> (42, 253.7735) projected
  line L730 (14.5, 258.1229) -> (19.5, 255.2361) projected
  line L731 (19.5, 255.2361) -> (24.5, 258.1229) projected
  line L732 (24.5, 258.1229) -> (24.5, 263.8964) projected
  line L733 (24.5, 263.8964) -> (19.5, 266.7831) projected
  line L734 (19.5, 266.7831) -> (14.5, 263.8964) projected
  line L735 (14.5, 263.8964) -> (14.5, 258.1229) projected
  line L736 (57, 279.7735) -> (52, 276.8868) projected
  line L737 (52, 276.8868) -> (52, 271.1132) projected
  line L738 (52, 271.1132) -> (57, 268.2265) projected
  line L739 (57, 268.2265) -> (62, 271.1132) projected
  line L740 (62, 271.1132) -> (62, 276.8868) projected
  line L741 (62, 276.8868) -> (57, 279.7735) projected
  line L742 (32, 302.8868) -> (27, 305.7735) projected
  line L743 (27, 305.7735) -> (22, 302.8868) projected
  line L744 (22, 302.8868) -> (22, 297.1132) projected
  line L745 (22, 297.1132) -> (27, 294.2265) projected
  line L746 (27, 294.2265) -> (32, 297.1132) projected
  line L747 (32, 297.1132) -> (32, 302.8868) projected
  line L748 (42, 305.7735) -> (37, 302.8868) projected
  line L749 (37, 302.8868) -> (37, 297.1132) projected
  line L750 (37, 297.1132) -> (42, 294.2265) projected
  line L751 (42, 294.2265) -> (47, 297.1132) projected
  line L752 (47, 297.1132) -> (47, 302.8868) projected
  line L753 (47, 302.8868) -> (42, 305.7735) projected
  line L754 (42, 331.7735) -> (37, 328.8868) projected
  line L755 (37, 328.8868) -> (37, 323.1132) projected
  line L756 (37, 323.1132) -> (42, 320.2265) projected
  line L757 (42, 320.2265) -> (47, 323.1132) projected
  line L758 (47, 323.1132) -> (47, 328.8868) projected
  line L759 (47, 328.8868) -> (42, 331.7735) projected
  line L760 (12, 357.7735) -> (7, 354.8868) projected
  line L761 (7, 354.8868) -> (7, 349.1132) projected
  line L762 (7, 349.1132) -> (12, 346.2265) projected
  line L763 (12, 346.2265) -> (17, 349.1132) projected
  line L764 (17, 349.1132) -> (17, 354.8868) projected
  line L765 (17, 354.8868) -> (12, 357.7735) projected
  line L766 (54.5, 341.8964) -> (49.5, 344.7831) projected
  line L767 (49.5, 344.7831) -> (44.5, 341.8964) projected
  line L768 (44.5, 341.8964) -> (44.5, 336.1229) projected
  line L769 (44.5, 336.1229) -> (49.5, 333.2361) projected
  line L770 (49.5, 333.2361) -> (54.5, 336.1229) projected
  line L771 (54.5, 336.1229) -> (54.5, 341.8964) projected
  line L772 (19.5, 359.2361) -> (24.5, 362.1229) projected
  line L773 (24.5, 362.1229) -> (24.5, 367.8964) projected
  line L774 (24.5, 367.8964) -> (19.5, 370.7831) projected
  line L775 (19.5, 370.7831) -> (14.5, 367.8964) projected
  line L776 (14.5, 367.8964) -> (14.5, 362.1229) projected
  line L777 (14.5, 362.1229) -> (19.5, 359.2361) projected
  line L778 (62, 380.8868) -> (57, 383.7735) projected
  line L779 (57, 383.7735) -> (52, 380.8868) projected
  line L780 (52, 380.8868) -> (52, 375.1132) projected
  line L781 (52, 375.1132) -> (57, 372.2265) projected
  line L782 (57, 372.2265) -> (62, 375.1132) projected
  line L783 (62, 375.1132) -> (62, 380.8868) projected
  point P0 (0, 0)
extrude "Extrusion1" add sketch "Sketch1" along normal blind 2 contours L0 L1 L2 L3 | A10 | A11 | A12 | A13 | L9 L8 L7 L6 L5 L4 | L15 L14 L13 L12 L11 L10 | L21 L20 L19 L18 L17 L16 | L27 L26 L25 L24 L23 L22 | L33 L32 L31 L30 L29 L28 | L39 L38 L37 L36 L35 L34 | L45 L44 L43 L42 L41 L40 | L51 L50 L49 L48 L47 L46 | L57 L56 L55 L54 L53 L52 | L63 L62 L61 L60 L59 L58 | L69 L68 L67 L66 L65 L64 | L75 L74 L73 L72 L71 L70 | L81 L80 L79 L78 L77 L76 | L87 L86 L85 L84 L83 L82 | L93 L92 L91 L90 L89 L88 | L99 L98 L97 L96 L95 L94 | L105 L104 L103 L102 L101 L100 | L111 L110 L109 L108 L107 L106 | L117 L116 L115 L114 L113 L112 | L123 L122 L121 L120 L119 L118 | L129 L128 L127 L126 L125 L124 | L135 L134 L133 L132 L131 L130 | L141 L140 L139 L138 L137 L136 | L147 L146 L145 L144 L143 L142 | L153 L152 L151 L150 L149 L148 | L159 L158 L157 L156 L155 L154 | L165 L164 L163 L162 L161 L160 | L171 L170 L169 L168 L167 L166 | L177 L176 L175 L174 L173 L172 | L183 L182 L181 L180 L179 L178 | L189 L188 L187 L186 L185 L184 | L195 L194 L193 L192 L191 L190 | L201 L200 L199 L198 L197 L196 | L207 L206 L205 L204 L203 L202 | L213 L212 L211 L210 L209 L208 | L219 L218 L217 L216 L215 L214 | L225 L224 L223 L222 L221 L220 | L231 L230 L229 L228 L227 L226 | L237 L236 L235 L234 L233 L232 | L243 L242 L241 L240 L239 L238 | L249 L248 L247 L246 L245 L244 | L255 L254 L253 L252 L251 L250 | L261 L260 L259 L258 L257 L256 | L267 L266 L265 L264 L263 L262 | L273 L272 L271 L270 L269 L268 | L279 L278 L277 L276 L275 L274 | L285 L284 L283 L282 L281 L280 | L291 L290 L289 L288 L287 L286 | L297 L296 L295 L294 L293 L292 | L303 L302 L301 L300 L299 L298 | L309 L308 L307 L306 L305 L304 | L315 L314 L313 L312 L311 L310 | L321 L320 L319 L318 L317 L316 | L327 L326 L325 L324 L323 L322 | L333 L332 L331 L330 L329 L328 | L339 L338 L337 L336 L335 L334 | L345 L344 L343 L342 L341 L340 | L351 L350 L349 L348 L347 L346 | L357 L356 L355 L354 L353 L352 | L363 L362 L361 L360 L359 L358 | L369 L368 L367 L366 L365 L364 | L375 L374 L373 L372 L371 L370 | L381 L380 L379 L378 L377 L376 | L387 L386 L385 L384 L383 L382 | L393 L392 L391 L390 L389 L388 | L399 L398 L397 L396 L395 L394 | L405 L404 L403 L402 L401 L400 | L411 L410 L409 L408 L407 L406 | L417 L416 L415 L414 L413 L412 | L423 L422 L421 L420 L419 L418 | L429 L428 L427 L426 L425 L424 | L435 L434 L433 L432 L431 L430 | L441 L440 L439 L438 L437 L436 | L447 L446 L445 L444 L443 L442 | L453 L452 L451 L450 L449 L448 | L459 L458 L457 L456 L455 L454 | L465 L464 L463 L462 L461 L460 | L471 L470 L469 L468 L467 L466 | L477 L476 L475 L474 L473 L472 | L483 L482 L481 L480 L479 L478 | L489 L488 L487 L486 L485 L484 | L495 L494 L493 L492 L491 L490 | L501 L500 L499 L498 L497 L496 | L507 L506 L505 L504 L503 L502 | L513 L512 L511 L510 L509 L508 | L519 L518 L517 L516 L515 L514 | L525 L524 L523 L522 L521 L520 | L531 L530 L529 L528 L527 L526 | L537 L536 L535 L534 L533 L532 | L543 L542 L541 L540 L539 L538 | L549 L548 L547 L546 L545 L544 | L555 L554 L553 L552 L551 L550 | L561 L560 L559 L558 L557 L556 | L567 L566 L565 L564 L563 L562 | L573 L572 L571 L570 L569 L568 | L579 L578 L577 L576 L575 L574 | L585 L584 L583 L582 L581 L580 | L591 L590 L589 L588 L587 L586 | L597 L596 L595 L594 L593 L592 | L603 L602 L601 L600 L599 L598 | L609 L608 L607 L606 L605 L604 | L615 L614 L613 L612 L611 L610 | L621 L620 L619 L618 L617 L616 | L627 L626 L625 L624 L623 L622 | L633 L632 L631 L630 L629 L628 | L639 L638 L637 L636 L635 L634 | L645 L644 L643 L642 L641 L640 | L651 L650 L649 L648 L647 L646 | L657 L656 L655 L654 L653 L652 | L663 L662 L661 L660 L659 L658 | L669 L668 L667 L666 L665 L664 | L675 L674 L673 L672 L671 L670 | L681 L680 L679 L678 L677 L676 | L687 L686 L685 L684 L683 L682 | L693 L692 L691 L690 L689 L688 | L699 L698 L697 L696 L695 L694 | L705 L704 L703 L702 L701 L700 | L711 L710 L709 L708 L707 L706 | L717 L716 L715 L714 L713 L712 | L723 L722 L721 L720 L719 L718 | L729 L728 L727 L726 L725 L724 | L735 L734 L733 L732 L731 L730 | L741 L740 L739 L738 L737 L736 | L747 L746 L745 L744 L743 L742 | L753 L752 L751 L750 L749 L748 | L759 L758 L757 L756 L755 L754 | L765 L764 L763 L762 L761 L760 | L771 L770 L769 L768 L767 L766 | L777 L776 L775 L774 L773 L772 | L783 L782 L781 L780 L779 L778
sketch "Sketch2" plane through (0, 0, 0) normal (-1, 0, 0) x (0, 0, 1)
  line L0 (411, -15) -> (-123, -15) projected
  line L1 (411, 465) -> (411, -15) projected
  line L2 (-123, 465) -> (411, 465) projected
  line L3 (-123, -15) -> (-123, 465) projected
  circle A0 centre (-113.5, 50) radius 1.75 projected
  circle A1 centre (-21, 457.5) radius 1.75 projected
  circle A2 centre (144, 457.5) radius 1.75 projected
  circle A3 centre (309, -7.5) radius 1.75 projected
  circle A4 centre (144, -7.5) radius 1.75 projected
  circle A5 centre (-21, -7.5) radius 1.75 projected
  circle A6 centre (401.5, 400) radius 1.75 projected
  circle A7 centre (401.5, 50) radius 1.75 projected
  circle A8 centre (-113.5, 400) radius 1.75 projected
  circle A9 centre (309, 457.5) radius 1.75 projected
  line L4 (-73, 425) -> (361, 425)
  line L5 (361, 425) -> (361, 92)
  line L6 (361, 92) -> (-73, 92)
  line L7 (-73, 92) -> (-73, 425)
  point P0 (0, 0)
  dimension "d2" = 50
  dimension "d3" = 50
  dimension "d4" = 40
  dimension "d5" = 107
  constraints: 8 end point, 2 parallel, 1 horizontal, 1 perpendicular
  measures "d2" distance between parallel lines of L3 L7
  measures "d3" distance between parallel lines of L1 L5
  measures "d4" distance between parallel lines of L2 L4
  measures "d5" distance between parallel lines of L0 L6
extrude "Extrusion2" cut sketch "Sketch2" against normal blind 2 contours L4 L5 L6 L7
chamfer "Chamfer1" distance 30 angle 45 2 edges at (1, 92, -73) (1, 92, 361)
sketch "Sketch3" plane through (0, 0, 0) normal (-1, 0, 0) x (0, 0, 1)
  line L0 (361, 425) -> (361, 122) projected
  line L1 (331, 92) -> (361, 122) projected
  line L2 (331, 92) -> (-43, 92) projected
  line L3 (-73, 122) -> (-43, 92) projected
  line L4 (-73, 122) -> (-73, 425) projected
  line L5 (-73, 425) -> (361, 425) projected
  line L6 (411, -15) -> (-123, -15) projected
  line L7 (411, 465) -> (411, -15) projected
  line L8 (-123, 465) -> (411, 465) projected
  line L9 (-123, -15) -> (-123, 465) projected
  circle A0 centre (-113.5, 50) radius 1.75 projected
  circle A1 centre (-21, 457.5) radius 1.75 projected
  circle A2 centre (144, 457.5) radius 1.75 projected
  circle A3 centre (309, -7.5) radius 1.75 projected
  circle A4 centre (144, -7.5) radius 1.75 projected
  circle A5 centre (-21, -7.5) radius 1.75 projected
  circle A6 centre (401.5, 400) radius 1.75 projected
  circle A7 centre (401.5, 50) radius 1.75 projected
  circle A8 centre (-113.5, 400) radius 1.75 projected
  circle A9 centre (309, 457.5) radius 1.75 projected
  circle A10 centre (311, 45) radius 11.5
  point P0 (0, 0)
  dimension "d11" = 23
  dimension "d12" = 60
  dimension "d13" = 100
  constraints: 1 centre point
  measures "d11" diameter of A10
  measures "d12" distance from line of L6 A10.centre
  measures "d13" distance from line of L7 A10.centre
extrude "Extrusion3" cut sketch "Sketch3" against normal through all contours A10
equation "\"d3\" = d2"
body "Solid1"
